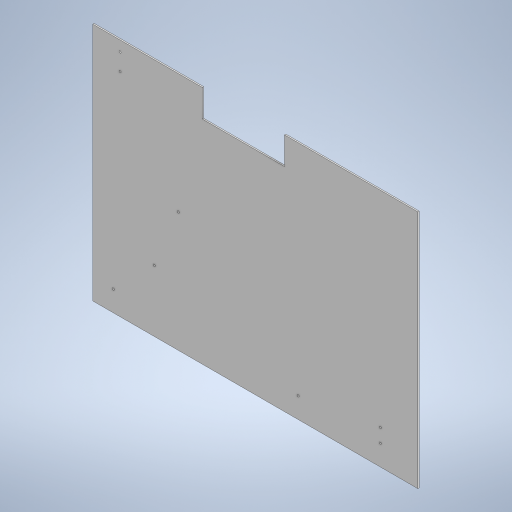
# Autodesk Inventor part: Cover
Saved by Autodesk Inventor 2023 (Build 270158000, 158)
## iProperties
Created: 2023-05-19
Part Number: Cover
Material: Generic
Document SubType Name: Modeling
Designer: Nathann
Density: 1 g/cm^3
Appearance: Default
Author: Nathann
Autodesk Inventor part; units mm, degrees
ref_plane "YZ Plane" through (0, 0, 0) normal (1, 0, 0) x (0, 1, 0)
ref_plane "XZ Plane" through (0, 0, 0) normal (0, 1, 0) x (-1, 0, 0)
ref_plane "XY Plane" through (0, 0, 0) normal (0, 0, 1) x (1, 0, 0)
sketch "Sketch1" plane through (0, 0, 0) normal (0, 0, 1) x (1, 0, 0)
  circle A0 centre (378.9358, -27.5) radius 1.5 projected
  circle A1 centre (378.9357, -47.5) radius 1.5 projected
  circle A2 centre (-1.0643, 232.5) radius 1.5 projected
  circle A3 centre (-1.0643, 257.5) radius 1.5 projected
  arc A4 (294.7595, 91.2473) -> (294.7595, 103.7527) centre (283.9357, 97.5) ccw projected
  arc A5 (269.1765, 26.4014) -> (294.7595, 91.2473) centre (183.9357, 97.5) ccw projected
  line L0 (269.1765, 26.4014) -> (346.8159, -51.238) projected
  line L1 (346.8159, -51.238) -> (340.2309, -57.3809) projected
  line L2 (340.2309, -57.3809) -> (198.7673, 84.0827) projected
  arc A6 (198.7673, 84.0827) -> (203.2542, 92.3236) centre (183.9357, 97.5) ccw projected
  line L3 (203.2542, 92.3236) -> (268.4665, 27.1114) projected
  arc A7 (268.4665, 27.1114) -> (293.6545, 89.639) centre (183.9357, 97.5) ccw projected
  arc A8 (293.6545, 105.361) -> (293.6545, 89.639) centre (283.9357, 97.5) ccw projected
  arc A9 (293.6545, 105.361) -> (268.4665, 167.8886) centre (183.9357, 97.5) ccw projected
  line L4 (268.4665, 167.8886) -> (203.2542, 102.6764) projected
  arc A10 (203.2542, 102.6764) -> (198.7673, 110.9173) centre (183.9357, 97.5) ccw projected
  line L5 (198.7673, 110.9173) -> (340.2063, 252.3564) projected
  line L6 (340.2063, 252.3564) -> (346.5703, 245.9924) projected
  line L7 (346.5703, 245.9924) -> (269.1765, 168.5986) projected
  arc A11 (294.7595, 103.7527) -> (269.1765, 168.5986) centre (183.9357, 97.5) ccw projected
  circle A12 centre (83.9357, 97.5) radius 1.5 projected
  line L8 (238.9357, 272.5) -> (238.9357, 232.5) projected
  line L9 (238.9357, 232.5) -> (118.9357, 232.5) projected
  line L10 (118.9357, 232.5) -> (118.9357, 272.5) projected
  line L11 (118.9357, 272.5) -> (-41.0643, 272.5) projected
  line L12 (-41.0643, 272.5) -> (-41.0643, -77.5) projected
  line L13 (-41.0643, -77.5) -> (433.9357, -77.5) projected
  line L14 (433.9357, -77.5) -> (433.9357, 272.5) projected
  line L15 (433.9357, 272.5) -> (238.9357, 272.5) projected
  circle A13 centre (-11.0643, -47.5) radius 1.5 projected
  circle A14 centre (48.9357, 12.5) radius 1.5 projected
  circle A15 centre (258.9357, -47.5) radius 1.5 projected
  line L16 (106.154, 175.2817) -> (169.7936, 111.6421) projected
  arc A16 (169.7936, 111.6421) -> (165.6054, 105.5) centre (183.9357, 97.5) ccw projected
  line L17 (165.6054, 105.5) -> (74.227, 105.5) projected
  arc A17 (74.227, 105.5) -> (74.227, 89.5) centre (183.9357, 97.5) ccw projected
  line L18 (74.227, 89.5) -> (165.6054, 89.5) projected
  arc A18 (165.6054, 89.5) -> (169.7936, 83.3579) centre (183.9357, 97.5) ccw projected
  line L19 (169.7936, 83.3579) -> (106.154, 19.7183) projected
  arc A19 (106.154, 19.7183) -> (254.3243, 12.9693) centre (183.9357, 97.5) ccw projected
  line L20 (254.3243, 12.9693) -> (189.1121, 78.1815) projected
  arc A20 (189.1121, 78.1815) -> (197.3531, 82.6684) centre (183.9357, 97.5) ccw projected
  line L21 (197.3531, 82.6684) -> (338.7675, -58.746) projected
  line L22 (338.7675, -58.746) -> (332.1825, -64.8889) projected
  line L23 (332.1825, -64.8889) -> (255.0343, 12.2592) projected
  arc A21 (255.0343, 182.7408) -> (255.0343, 12.2592) centre (183.9357, 97.5) ccw projected
  line L24 (255.0343, 182.7408) -> (332.4281, 260.1346) projected
  line L25 (332.4281, 260.1346) -> (338.7921, 253.7706) projected
  line L26 (338.7921, 253.7706) -> (197.3531, 112.3316) projected
  arc A22 (197.3531, 112.3316) -> (189.1121, 116.8185) centre (183.9357, 97.5) ccw projected
  line L27 (189.1121, 116.8185) -> (254.3243, 182.0307) projected
  arc A23 (254.3243, 182.0307) -> (106.154, 175.2817) centre (183.9357, 97.5) ccw projected
  point P0 (0, 0)
extrude "Extrusion1" add sketch "Sketch1" along normal blind 2 contours A5 L0 L1 L2 A6 L3 A7 A8 A9 L4 A10 L5 L6 L7 A11 A4 | L15 L14 L13 L12 L11 L10 L9 L8 | L16 A16 L17 A17 L18 A18 L19 A19 L20 A20 L21 L22 L23 A21 L24 L25 L26 A22 L27 A23
body "Solid1"
